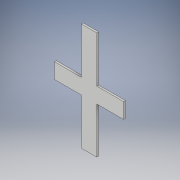
# Autodesk Inventor part: backplatelift
Saved by Autodesk Inventor 2017 (Build 210142000, 142)
## iProperties
Created: 2017-05-30
Part Number: backplatelift
Material: Generic
Document SubType Name: Modeling
Designer: User
Density: 1 g/cm^3
Appearance: Default
Author: User
Autodesk Inventor part; units mm, degrees
ref_plane "YZ Plane" through (0, 0, 0) normal (1, 0, 0) x (0, 1, 0)
ref_plane "XZ Plane" through (0, 0, 0) normal (0, 1, 0) x (-1, 0, 0)
ref_plane "XY Plane" through (0, 0, 0) normal (0, 0, 1) x (1, 0, 0)
sketch "Sketch1" plane through (0, 0, 0) normal (0, 0, 1) x (1, 0, 0)
  line L0 (0, 0) -> (50.8, 0)
  line L1 (50.8, 0) -> (50.8, 355.6)
  line L2 (50.8, 355.6) -> (0, 355.6)
  line L3 (0, 355.6) -> (0, 0)
  dimension "d0" = 50.8
  dimension "d1" = 355.6
  constraints: 8 end point, 2 parallel, 1 horizontal, 1 perpendicular
  measures "d0" distance of L2.end L1.end
  measures "d1" distance of L1.end L0.end
extrude "Extrusion1" add sketch "Sketch1" along normal blind 6.35
sketch "Sketch2" plane through (0, 0, 6.35) normal (0, 0, 1) x (1, 0, 0)
  line L0 (50.8, 0) -> (50.8, 355.6) projected
  line L1 (50.8, 203.2) -> (139.7, 203.2)
  line L2 (139.7, 203.2) -> (139.7, 152.4)
  line L3 (139.7, 152.4) -> (50.8, 152.4)
  line L4 (50.8, 152.4) -> (50.8, 203.2)
  line L5 (0, 203.2) -> (-88.9, 203.2)
  line L6 (-88.9, 203.2) -> (-88.9, 152.4)
  line L7 (-88.9, 152.4) -> (0, 152.4)
  line L8 (0, 152.4) -> (0, 203.2)
  point P0 (0, 0)
  point P1 (50.8, 152.4)
  constraints: 16 end point, 4 parallel, 2 horizontal, 2 perpendicular, 2 point on line
extrude "Extrusion2" add sketch "Sketch2" against normal blind 6.35
body "Solid1"
